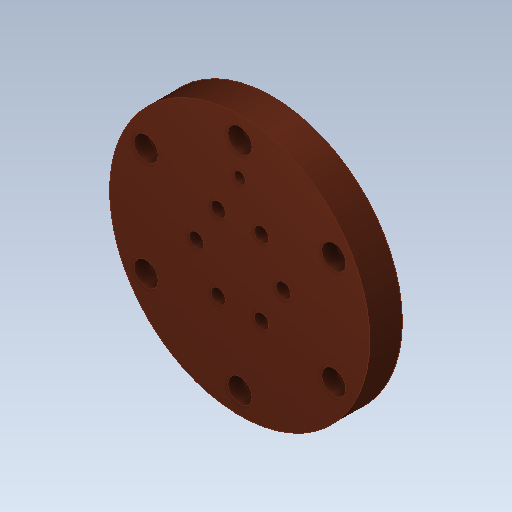
# Autodesk Inventor part: base_connector
Saved by Autodesk Inventor 2020.5 (Build 245400000, 400)
## iProperties
Created: 2018-08-22
Part Number: base_connector
Material: Copper
Document SubType Name: Modeling
Designer: Q
Density: 8.94 g/cm^3
Appearance: Copper - Satin
Mass: 1417.21 g
Surface Area: 323.134 cm^2
Volume: 158.525 cm^3
Author: Q
Autodesk Inventor part; units mm, degrees
ref_plane "YZ Plane" through (0, 0, 0) normal (1, 0, 0) x (0, 1, 0)
ref_plane "XZ Plane" through (0, 0, 0) normal (0, 1, 0) x (-1, 0, 0)
ref_plane "Work Plane2" through (0, 0, 0) normal (0, 0, 1) x (1, 0, 0)
sketch "Sketch26" plane through (0, 0, 0) normal (0, 0, 1) x (1, 0, 0)
  circle A0 centre (0, 0) radius 60 projected
  point P0 (0, 0)
extrude "Extrusion12" add sketch "Sketch26" along normal blind 15
sketch "Sketch28" plane through (0, 0, 0) normal (0, 0, -1) x (-1, 0, 0)
  circle A0 centre (0, 0) radius 30 projected
  circle A1 centre (0, 0) radius 20 construction
  point P0 (0, 0)
  point P1 (20, 0)
  dimension "d225" = 40
  constraints: 1 coincident, 1 horizontal alignment, 2 other
hole "Hole13" at (-20, 0, 0) direction (0, 0, 1) diameter 6.6 end through all counterbore diameter 11 counterbore depth 6.8 clearance for "Socket Head Cap Screw ISO 4762" size "M6" standard "ISO"
pattern_circular "Circular Pattern10" count 6 over 360 about axis through (0, 0, 0) along (0, 0, 1) of "Hole13"
sketch "Sketch29" plane through (0, 0, 15) normal (0, 0, 1) x (1, 0, 0)
  circle A0 centre (-43.3013, 25) radius 2.4585 projected
  circle A1 centre (-43.3013, -25) radius 2.4585 projected
  point P0 (0, 0)
  point P1 (-43.0428, -24.2502)
  point P2 (-40.9021, -15.0744)
hole "Hole14" at (-43.3013, 25, 15) direction (0, 0, -1) diameter 6.6 depth 17.1 counterbore diameter 11 counterbore depth 6.8 clearance for "Socket Head Cap Screw ISO 4762" size "M6" standard "ISO"
pattern_circular "Circular Pattern11" count 6 over 360 about axis through (0, 0, 0) along (0, 0, 1) of "Hole14"
sketch "Sketch30" plane through (0, 0, 0) normal (0, 0, -1) x (-1, 0, 0)
  circle A0 centre (0, 35) radius 2.067 construction
  circle A1 centre (0, 35) radius 2.5
  point P0 (0, 0)
  dimension "d248" = 5
  constraints: 1 centre point, 1 coincident
  measures "d248" diameter of A1
extrude "Extrusion13" cut sketch "Sketch30" against normal up to next
body "Solid2"
